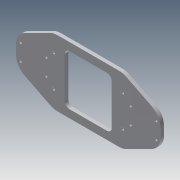
# Autodesk Inventor part: VatPlate
Saved by Autodesk Inventor 2014 (Build 180170000, 170)
## iProperties
Created: 2014-08-10
Part Number: VatPlate
Material: Generic
Document SubType Name: Modeling
Designer: Peele
Density: 1 g/cm^3
Appearance: White
Author: Peele
Autodesk Inventor part; units mm, degrees
ref_plane "YZ Plane" through (0, 0, 0) normal (1, 0, 0) x (0, 1, 0)
ref_plane "XZ Plane" through (0, 0, 0) normal (0, 1, 0) x (-1, 0, 0)
ref_plane "XY Plane" through (0, 0, 0) normal (0, 0, 1) x (1, 0, 0)
sketch "Sketch1" plane through (0, 0, 0) normal (0, 1, 0) x (-1, 0, 0)
  line L0 (-115, -52.5) -> (115, -52.5)
  line L1 (115, -52.5) -> (115, 52.5)
  line L2 (115, 52.5) -> (-115, 52.5)
  line L3 (-115, 52.5) -> (-115, -52.5)
  line L4 (-115, -52.5) -> (115, 52.5) construction
  line L5 (115, -52.5) -> (-115, 52.5) construction
  line L6 (-108, 13) -> (-67, 13) construction
  line L7 (-67, 13) -> (-67, -13) construction
  line L8 (-67, -13) -> (-108, -13) construction
  line L9 (-108, -13) -> (-108, 13) construction
  line L10 (-108, 13) -> (-67, -13) construction
  line L11 (-67, 13) -> (-108, -13) construction
  line L12 (67, 13) -> (108, 13) construction
  line L13 (108, 13) -> (108, -13) construction
  line L14 (108, -13) -> (67, -13) construction
  line L15 (67, -13) -> (67, 13) construction
  line L16 (67, 13) -> (108, -13) construction
  line L17 (108, 13) -> (67, -13) construction
  circle A0 centre (-67, 13) radius 2
  circle A1 centre (-67, -13) radius 2
  circle A2 centre (-108, -13) radius 2
  circle A3 centre (-108, 13) radius 2
  circle A4 centre (67, 13) radius 2
  circle A5 centre (108, 13) radius 2
  circle A6 centre (108, -13) radius 2
  circle A7 centre (67, -13) radius 2
  line L18 (-37.5, -40) -> (37.5, -40)
  line L19 (37.5, -40) -> (37.5, 40)
  line L20 (37.5, 40) -> (-37.5, 40)
  line L21 (-37.5, 40) -> (-37.5, -40)
  line L22 (-37.5, -40) -> (37.5, 40) construction
  line L23 (37.5, -40) -> (-37.5, 40) construction
  point P0 (0, 0)
  point P1 (-87.5, 0)
  point P2 (87.5, 0)
  dimension "d0" = 105
  dimension "d3" = 26
  dimension "d4" = 41
  dimension "d5" = 175
  dimension "d6" = 87.5
  dimension "d7" = 230
  dimension "d8" = 4
  dimension "d9" = 80
  dimension "d10" = 75
  constraints: 48 end point, 9 midpoint, 8 centre point, 8 coincident, 8 parallel, 7 equal radius, 4 horizontal, 4 perpendicular, 2 equal length, 1 collinear, 1 horizontal alignment
  measures "d0" distance of L2.end L0.start
  measures "d3" distance of L8.end L6.start
  measures "d4" distance of L7.end L8.end
  measures "d5" distance of point (87.5, 0) point (-87.5, 0)
  measures "d6" distance of point (-87.5, 0) point (0, 0)
  measures "d7" distance of L1.end L2.end
  measures "d8" diameter of A3
  measures "d9" distance of L20.end L18.start
  measures "d10" distance of L19.end L20.end
extrude "Extrusion1" add sketch "Sketch1" along normal blind 5.588
sketch "Sketch2" plane through (0, 0, 0) normal (0, -1, 0) x (1, 0, 0)
  line L0 (115, -52.5) -> (-115, -52.5) projected
  line L1 (115, 52.5) -> (115, -52.5) projected
  line L2 (-115, 52.5) -> (115, 52.5) projected
  line L3 (-115, -52.5) -> (-115, 52.5) projected
  line L4 (-115, 52.5) -> (-115, 22.5)
  line L5 (-115, 22.5) -> (-55, 52.5)
  line L6 (-55, 52.5) -> (-115, 52.5)
  line L7 (-115, -22.5) -> (-115, -52.5)
  line L8 (-115, -52.5) -> (-55, -52.5)
  line L9 (-115, -22.5) -> (-55, -52.5)
  line L10 (55, 52.5) -> (115, 22.5)
  line L11 (115, 22.5) -> (115, 52.5)
  line L12 (115, 52.5) -> (55, 52.5)
  line L13 (115, -22.5) -> (115, -52.5)
  line L14 (115, -52.5) -> (55, -52.5)
  line L15 (55, -52.5) -> (115, -22.5)
  point P0 (0, 0)
  dimension "d13" = 60
  dimension "d14" = 30
  constraints: 25 end point, 8 point on line, 3 collinear, 3 equal length, 2 horizontal alignment, 2 perpendicular, 2 vertical alignment
  measures "d13" distance of L5.end L2.start
  measures "d14" distance of L2.start L4.end
extrude "Extrusion2" cut sketch "Sketch2" against normal blind 10 contours L0 L15 L1 | L0 L3 L9 | L10 L2 L1 | L3 L2 L5
fillet "Fillet1" radius 25 8 edges at (-55, 2.794, -52.5) (-115, 2.794, -22.5) (55, 2.794, -52.5) (115, 2.794, -22.5) (115, 2.794, 22.5) (55, 2.794, 52.5) (-55, 2.794, 52.5) (-115, 2.794, 22.5)
sketch "Sketch4" plane through (0, 0, 0) normal (0, -1, 0) x (1, 0, 0)
  line L0 (55, -25) -> (-55, -25) construction
  line L1 (-55, -25) -> (-55, 25) construction
  line L2 (-55, 25) -> (55, 25) construction
  line L3 (55, 25) -> (55, -25) construction
  line L4 (55, -25) -> (-55, 25) construction
  line L5 (-55, -25) -> (55, 25) construction
  circle A0 centre (-55, 25) radius 2
  circle A1 centre (-55, -25) radius 2
  circle A2 centre (55, -25) radius 2
  circle A3 centre (55, 25) radius 2
  point P0 (0, 0)
  dimension "d18" = 4
  dimension "d20" = 50
  dimension "d23" = 110
  constraints: 12 end point, 4 centre point, 4 coincident, 3 equal radius, 2 midpoint, 2 parallel, 1 horizontal, 1 perpendicular
  measures "d18" diameter of A0
  measures "d20" distance of L0.end L1.end
  measures "d23" distance of L1.end L2.end
extrude "Extrusion3" cut sketch "Sketch4" against normal blind 10
fillet "Fillet2" radius 8 4 edges at (-37.5, 2.794, 40) (37.5, 2.794, 40) (-37.5, 2.794, -40) (37.5, 2.794, -40)
equation "\"d6\" = 0.5 * d5"
body "Solid1"
